MachinedHolder_v26 (Autodesk Fusion 360 design; units mm, degrees)
Autodesk Fusion 360 part; units mm, degrees
sketch "Sketch1" plane through (0, 0, 0) normal (0, 0, 1) x (1, 0, 0)
  circle A0 centre (0, 0) radius 19.05
  circle A1 centre (0, 0) radius 17.4625
  circle A2 centre (0, 0) radius 9.525
  circle A3 centre (0, 0) radius 11.1125
  circle A4 centre (0, 0) radius 14.2875 construction
  line L0 (0, 0) -> (0, 19.05) construction
  line L1 (0, 0) -> (19.05, 0) construction
  circle A5 centre (4.445, 13.5785) radius 3.175
  line L2 (-3.175, 19.05) -> (3.175, 19.05) construction
  line L3 (3.175, 19.05) -> (3.175, 8.9803) construction
  line L4 (3.175, 8.9803) -> (-3.175, 8.9803) construction
  line L5 (-3.175, 8.9803) -> (-3.175, 19.05) construction
  circle A6 centre (4.445, 13.5785) radius 1.27 construction
  line L6 (0, 13.09) -> (2.1968, 10.8932)
  line L7 (0, 0) -> (4.6567, 16.8302) construction
  arc A7 (4.6567, 16.8302) -> (2.9633, 10.7101) centre (3.81, 13.7701) ccw
  line L8 (0, 13.09) -> (-2.1968, 10.8932)
  arc A8 (-2.9633, 10.7101) -> (-4.6567, 16.8302) centre (-3.81, 13.7701) ccw
  circle A9 centre (-4.445, 13.5785) radius 3.175
  circle A10 centre (-13.9818, -2.9397) radius 3.175
  arc A11 (-16.9037, -4.3823) -> (-10.7569, -2.7887) centre (-13.8303, -3.5855) ccw
  arc A12 (-7.7936, -7.9214) -> (-12.247, -12.4479) centre (-10.0203, -10.1846) ccw
  circle A13 centre (-9.5368, -10.6387) radius 3.175
  line L9 (-11.3363, -6.545) -> (-8.3354, -7.3491)
  line L10 (-11.3363, -6.545) -> (-10.5322, -3.5441)
  circle A14 centre (9.5368, -10.6387) radius 3.175
  arc A15 (12.247, -12.4479) -> (7.7936, -7.9214) centre (10.0203, -10.1846) ccw
  arc A16 (10.7569, -2.7887) -> (16.9037, -4.3823) centre (13.8303, -3.5855) ccw
  circle A17 centre (13.9818, -2.9397) radius 3.175
  line L11 (11.3363, -6.545) -> (10.5322, -3.5441)
  line L12 (11.3363, -6.545) -> (8.3354, -7.3491)
  arc A18 (2.9633, -10.7101) -> (4.6567, -16.8302) centre (3.81, -13.7701) ccw
  line L13 (0, -13.09) -> (2.1968, -10.8932)
  line L14 (0, -13.09) -> (-2.1968, -10.8932)
  arc A19 (-4.6567, -16.8302) -> (-2.9633, -10.7101) centre (-3.81, -13.7701) ccw
  line L15 (4.445, 13.5785) -> (10.2849, 9.9174) construction
  line L16 (10.2849, 9.9174) -> (13.7311, 3.9483) construction
  line L17 (13.7311, 3.9483) -> (13.9818, -2.9397) construction
  circle A20 centre (0, 11.0017) radius 1.4767 construction
  line L18 (0.6748, -14.2716) -> (3.9169, -13.7401) construction
  line L19 (6.9518, -12.4822) -> (3.9169, -13.7401) construction
  line L20 (0, 0) -> (-16.4978, 9.525) construction
  line L21 (0, 0) -> (-9.525, -16.4978) construction
  line L22 (-4.445, 13.5785) -> (-13.9818, -2.9397) construction
  point P0 (0, 8.9803)
  point P1 (0, 11.1125)
  point P2 (13.7311, 3.9483)
  point P3 (10.2849, 9.9174)
  point P4 (-10.2849, 9.9174)
  point P5 (-13.7311, 3.9483)
  point P6 (0, 11.0017)
  point P7 (0, -11.0017)
  point P8 (-9.5277, -5.5008)
  point P9 (9.5277, -5.5008)
  point P10 (3.9169, -13.7401)
  point P11 (-3.9169, -13.7401)
  point P12 (-9.2134, 5.3194)
  dimension "d1" = 38.1
  dimension "d2" = 34.925
  dimension "d3" = 19.05
  dimension "d4" = 22.225
  dimension "d5" = 28.575
  dimension "d6" = 6.35
  dimension "d7" = 2.54
  dimension "d8" = 6.35
  dimension "d9" = 45
  dimension "d10" = 3.81
  dimension "d12" = 360
  dimension "d14" = 360
  constraint coincident A0.centre A1.centre
  constraint concentric A0 A1
  constraint concentric A0 A2
  constraint concentric A2 A4
  constraint coincident A0 L0.end
  constraint vertical L0
  constraint coincident A0 L1.end
  constraint perpendicular L0 L1
  constraint coincident A4 A5.centre
  constraint horizontal L2
  constraint vertical L3
  constraint horizontal L4
  constraint vertical L5
  constraint coincident A2 L3.end
  constraint concentric A5 A6
  constraint tangent L3 A6
  constraint midpoint L4 P0
  constraint coincident L0 P0
  constraint tangent A0 L2
  constraint coincident L0 L6.start
  constraint coincident A3 L6.end
  constraint coincident A3 P1
  constraint coincident L0 P1
  constraint coincident A1 L7.end
  constraint coincident A3 A7.end
  constraint coincident L7 A7.end
  constraint coincident L7 A7.centre
  constraint tangent L6 A7
  constraint symmetric L0 A5 A9
  constraint symmetric L0 L6.start L8.start
  constraint symmetric L0 L6.end L8.end
  constraint symmetric L0 L7.end A8.end
  constraint symmetric L0 A7.end A8.start
  constraint symmetric L0 A7 A8
  constraint symmetric L1 L6.start L13.start
  constraint symmetric L1 L6.end L13.end
  constraint symmetric L1 L7.end A18.end
  constraint symmetric L1 A7.end A18.start
  constraint symmetric L1 A7 A18
  constraint symmetric L1 L8.end L14.end
  constraint symmetric L1 A8.end A19.start
  constraint symmetric L1 A8.start A19.end
  constraint symmetric L1 A8 A19
  constraint coincident A5.centre A6.centre
  constraint coincident A4 P3
  constraint coincident A4 P2
  constraint coincident A17.centre L17.end
  constraint coincident P2 L16.end
  constraint coincident P3 L15.end
  constraint equal L15 L16
  constraint equal L16 L17
  constraint symmetric L0 P2 P5
  constraint symmetric L0 P3 P4
  constraint tangent L6 A20
  constraint tangent L8 A20
  constraint tangent A2 A20
  constraint coincident P6 A20.centre
  constraint symmetric L1 P6 P7
  constraint coincident A4 L18.start
  constraint coincident A18 L18.start
  constraint coincident A4 P10
  constraint coincident A14 L19.start
  constraint coincident A4 L19.start
  constraint coincident P10 L18.end
  constraint equal L18 L19
  constraint symmetric L0 P10 P11
  constraint coincident A0 L20.end
  constraint coincident A0 L21.end
  constraint perpendicular L20 L21
  constraint coincident A9.centre L22.start
  constraint coincident A10.centre L22.end
  constraint midpoint L22 P12
  constraint coincident L20 P12
  measures "d1" diameter of A0
  measures "d2" diameter of A1
  measures "d3" diameter of A2
  measures "d4" diameter of A3
  measures "d5" diameter of A4
  measures "d6" diameter of A5
  measures "d7" diameter of A6
  measures "d8" distance of L2.start L2.end
  measures "d9" angle of L0 L6
  measures "d10" distance of L0 A7.centre
extrude "Extrude1" add sketch "Sketch1" against normal blind 2.54 contours A0 | A1 L6 A7 L8 A8 | A1 A3 A5 A7 | A1 A3 A8 A9 | A1 A3 A5 A17 | A5 | A3 L6 L8 | A3 L6 A7 | A1 A3 A9 A10 | A9 | A3 L8 A8 | A3 | A1 A3 A10 A11 | A10 | A1 A3 A16 A17 | A17 | A1 A11 A12 L9 L10 | A1 A15 A16 L11 L12 | A1 A3 A12 A13 | A3 L9 L10 | A3 A11 L10 | A1 A3 A14 A15 | A3 A16 L11 | A3 L11 L12 | A1 A3 A13 A19 | A13 | A3 A12 L9 | A1 A3 A14 A18 | A14 | A3 A15 L12 | A1 A18 L13 L14 A19 | A3 L13 L14 | A3 L14 A19 | A3 A18 L13 makes body 1
extrude "Extrude2" add sketch "Sketch1" along normal blind 0.635 contours A0 | A3 L6 L8 | A3 | A3 L9 L10 | A3 L11 L12 | A3 L13 L14 bodies 1
hole "Hole1" at (4.445, 13.5785, 0) at (-4.445, 13.5785, 0) at (-10.2849, 9.9174, 0) at (-13.7311, 3.9483, 0) at (-13.9818, -2.9397, 0) at (-9.5368, -10.6387, 0) at (-3.9169, -13.7401, 0) at (3.9169, -13.7401, 0) at (9.5368, -10.6387, 0) at (13.9818, -2.9397, 0) at (13.7311, 3.9483, 0) at (10.2849, 9.9174, 0) direction (0, 0, -1) diameter 3.2639 end up to surface (2.54 mm away) bodies 1
move_face "OffsetFaces1" offset -0.254 13 faces at (2.1714, -17.327, 0.4233) (4.4845, -10.1674, 0.4233) (0.7323, -12.3577, 0.2117) (9.8748, 5.0968, 0.2117) (11.0682, -5.5447, 0.2117) (10.336, -6.813, 0.2117) (-0.7323, 12.3577, 0.2117) (-9.0581, 6.4372, 0.2117) (0.7323, 12.3577, 0.2117) (-10.336, -6.813, 0.2117) (-11.0682, -5.5447, 0.2117) (-5.3467, -9.7417, 0.4233) (-0.7323, -12.3577, 0.2117) on bodies 1
extrude "Extrude3" add sketch "Sketch1" along normal blind 3.175 separate body contours A1 A3 A5 A7 | A1 A3 A8 A9 | A1 A3 A5 A17 | A5 | A1 A3 A9 A10 | A9 | A1 A3 A10 A11 | A10 | A1 A3 A16 A17 | A17 | A1 A3 A12 A13 | A1 A3 A14 A15 | A1 A3 A13 A19 | A13 | A1 A3 A14 A18 | A14 makes body 2 at (15.0995, -2.5286, 3.175) makes body 3 at (3.0678, -14.5245, 0) makes body 4 at (-2.7528, 13.8183, 3.175) makes body 5 at (-10.6948, -9.1741, 0)
sketch "Sketch2" plane through (0, 0, 3.175) normal (0, 0, 1) x (-1, 0, 0)
  arc A0 (2.9633, -10.7101) -> (4.6567, -16.8302) centre (3.81, -13.7701) ccw
  arc A1 (4.6567, -16.8302) -> (16.9037, 4.3823) centre (0, 0) ccw
  arc A2 (16.9037, 4.3823) -> (10.7569, 2.7887) centre (13.8303, 3.5855) ccw
  arc A3 (2.9633, -10.7101) -> (10.7569, 2.7887) centre (0, 0) ccw
  circle A4 centre (-4.445, -13.5785) radius 3.175
  circle A5 centre (4.445, -13.5785) radius 3.175
  circle A6 centre (13.9818, 2.9397) radius 3.175
  circle A7 centre (9.5368, 10.6387) radius 3.175
  circle A8 centre (-9.5368, 10.6387) radius 3.175
  circle A9 centre (-13.9818, 2.9397) radius 3.175
  line L0 (-4.445, -16.7535) -> (-4.445, -10.4035)
  line L1 (4.445, -16.7535) -> (4.445, -10.1848)
  line L2 (13.9818, -0.2353) -> (13.9818, 6.1147)
  line L3 (9.5368, 7.4637) -> (9.5368, 13.8137)
  line L4 (-9.5368, 7.4637) -> (-9.5368, 13.8137)
  line L5 (-13.9818, 6.1147) -> (-13.9818, -0.2353)
  point P0 (10.2849, -9.9174)
  point P1 (13.7311, -3.9483)
  point P2 (3.9169, 13.7401)
  point P3 (-3.9169, 13.7401)
  point P4 (-10.2849, -9.9174)
  point P5 (-13.7311, -3.9483)
  point P6 (-4.445, -13.5785)
  point P7 (4.445, -13.5785)
  point P8 (13.9818, 2.9397)
  point P9 (9.5368, 10.6387)
  point P10 (-9.5368, 10.6387)
  point P11 (-13.9818, 2.9397)
  constraint coincident A4 L0.start
  constraint coincident A4 L0.end
  constraint vertical L0
  constraint coincident A5 L1.start
  constraint coincident A3 L1.end
  constraint parallel L0 L1
  constraint coincident A6 L2.start
  constraint coincident A6 L2.end
  constraint parallel L1 L2
  constraint coincident A7 L3.start
  constraint coincident A7 L3.end
  constraint parallel L2 L3
  constraint coincident A8 L4.end
  constraint parallel L3 L4
  constraint coincident A9 L5.start
  constraint coincident A9 L5.end
  constraint parallel L4 L5
  constraint coincident L0 P6
  constraint coincident L1 P7
  constraint coincident L2 P8
  constraint coincident L3 P9
  constraint coincident L4 P10
  constraint coincident L5 P11
  constraint coincident A8 L4.start
revolve "Revolve1" add sketch "Sketch2" angle 180 about axis through (-4.445, 16.7535, 3.175) along (0, 1, 0) contours A5 L1 picked at (6.1429, -14.5037) bodies 4
revolve "Revolve2" add sketch "Sketch2" angle 180 about axis through (-13.9818, 0.2353, 3.175) along (0, 1, 0) contours A6 L2 picked at (14.6749, 2.1399) bodies 4
revolve "Revolve3" add sketch "Sketch2" angle 180 about axis through (-9.5368, -7.4637, 3.175) along (0, 1, 0) contours A7 L3 picked at (10.5523, 10.9369) bodies 5
revolve "Revolve4" add sketch "Sketch2" angle 180 about axis through (4.445, 16.7535, 3.175) along (0, 1, 0) contours A4 L0 picked at (-3.1964, -12.9175) bodies 2
revolve "Revolve5" add sketch "Sketch2" angle 180 about axis through (13.9818, -6.1147, 3.175) along (0, 1, 0) contours A9 L5 picked at (-12.8157, 3.2271) bodies 2
revolve "Revolve6" add sketch "Sketch2" angle 180 about axis through (9.5368, -7.4637, 3.175) along (0, 1, 0) contours A8 L4 picked at (-8.2232, 10.9798) bodies 3
hole "Hole2" at (13.9818, -2.9397, 0) at (13.7311, 3.9483, 0) at (10.2849, 9.9174, 0) at (4.445, 13.5785, 0) at (-4.445, 13.5785, 0) at (-10.2849, 9.9174, 0) at (-13.7311, 3.9483, 0) at (-13.9818, -2.9397, 0) at (-9.5368, -10.6387, 0) at (9.5368, -10.6387, 0) at (3.9169, -13.7401, 0) at (-3.9169, -13.7401, 0) direction (0, 0, 1) diameter 2.2708 depth 6.35 tip angle 180 bodies 2 3 4 5
thread "Thread1" "ANSI Unified Screw Threads 0.112(#4) 4-40 UNC 2B" major diameter 2.8448 minor diameter 2.2708 pitch 0.635 angle 60 resizes the face on face at (-3.8038, -12.6104, 1.0583) on face at (-13.6181, 5.078, 1.0583) on face at (9.5934, -9.5047, 4.0934) on face at (-10.1718, 11.0471, 1.0583) on face at (4.0299, -12.6104, 1.0583) on face at (10.3979, 11.0471, 1.0583) on face at (-4.332, 14.7082, 2.0467) on face at (-9.4802, -9.5047, 4.0934) on face at (4.558, 14.7082, 2.0467) on face at (-13.9252, -1.8058, 4.0934) on face at (13.8442, 5.078, 1.0583) on face at (14.0384, -1.8058, 4.0934) on bodies 2 3 4 5
sketch "Sketch3" plane through (0, 0, -2.54) normal (0, 0, -1) x (1, 0, 0)
  circle A0 centre (13.7311, -3.9483) radius 1.6319
  circle A1 centre (9.5368, 10.6387) radius 1.6319
  circle A2 centre (-3.9169, 13.7401) radius 1.6319
  circle A3 centre (-13.9818, 2.9397) radius 1.6319
  circle A4 centre (-10.2849, -9.9174) radius 1.6319
  circle A5 centre (4.445, -13.5785) radius 1.6319
  circle A6 centre (-4.445, -13.5785) radius 1.6319
  circle A7 centre (-13.7311, -3.9483) radius 1.6319
  circle A8 centre (-9.5368, 10.6387) radius 1.6319
  circle A9 centre (3.9169, 13.7401) radius 1.6319
  circle A10 centre (13.9818, 2.9397) radius 1.6319
  circle A11 centre (10.2849, -9.9174) radius 1.6319
  circle A12 centre (0, 0) radius 9.525
  circle A13 centre (0, 0) radius 19.05
  point P0 (-9.5277, 5.5008)
  point P1 (0, 11.0017)
  point P2 (9.5277, 5.5008)
  point P3 (0, -11.0017)
hole "Hole3" at (0, 11.0017, -2.54) at (-9.5277, -5.5008, -2.54) at (9.5277, -5.5008, -2.54) direction (0, 0, 1) diameter 1.7831 depth 3.175 tip angle 180 bodies 1
thread "Thread2" "ANSI Unified Screw Threads 0.086(#2) 2-56 UNC 2B" major diameter 2.1844 minor diameter 1.7831 pitch 0.4536 angle 60 resizes the face on face at (9.6165, -4.6137, -1.4817) on face at (0.0888, 11.8888, -1.4817) on face at (-9.439, -4.6137, -1.4817) on bodies 1
move_face "OffsetFaces2" offset -0.127 1 faces at (-18.9553, 1.8968, -0.4233) on bodies 1
fillet "Fillet1" radius 1.778 8 edges at (-8.1951, -7.1237, 0.3175) (-2.0718, -10.659, 0.3175) (2.0718, -10.659, 0.3175) (8.1951, -7.1237, 0.3175) (10.2669, -3.5353, 0.3175) (2.0718, 10.659, 0.3175) (-2.0718, 10.659, 0.3175) (-10.2669, -3.5353, 0.3175) on bodies 1
copy_body "Body->Comp1" bodies 1 removing the originals makes body 6 in component "mainHolder"
copy_body "Body->Comp2" bodies 5 removing the originals makes body 7 in component "bottomLeft"
copy_body "Body->Comp3" bodies 2 removing the originals makes body 8 in component "topRight"
copy_body "Body->Comp4" bodies 3 removing the originals makes body 9 in component "bottomRight"
copy_body "Body->Comp5" bodies 4 removing the originals makes body 10 in component "topLeft"
ref_plane "WorkPlane1" through (6.35, 0, 0) normal (1, 0, 0) x (0, 1, 0)
component "mainHolder" placed x (1, 0, 0) y (0, 1, 0) z (0, 0, 1) at (0, 0, 0)
component "bottomLeft" placed x (1, 0, 0) y (0, 1, 0) z (0, 0, 1) at (0, 0, 0)
component "topRight" placed x (1, 0, 0) y (0, 1, 0) z (0, 0, 1) at (0, 0, 0)
component "bottomRight" placed x (1, 0, 0) y (0, 1, 0) z (0, 0, 1) at (0, 0, 0)
component "topLeft" placed x (1, 0, 0) y (0, 1, 0) z (0, 0, 1) at (0, 0, 0)
named bodies: "mainHolder", "topRight", "bottomRight", "topLeft", "bottomLeft"
